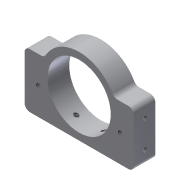
# Autodesk Inventor part: Motor Mount New - Estimated Dimensions
Saved by Autodesk Inventor 2013 (Build 170138000, 138)
## iProperties
Created: 2013-07-20
Part Number: Motor Mount New - Estimated Dimensions
Material: Aluminum 6061
Document SubType Name: Modeling
Designer: Nemo
Density: 1 g/cm^3
Author: Nemo
Autodesk Inventor part; units mm, degrees
ref_plane "YZ Plane" through (0, 0, 0) normal (1, 0, 0) x (0, 1, 0)
ref_plane "XZ Plane" through (0, 0, 0) normal (0, 1, 0) x (-1, 0, 0)
ref_plane "XY Plane" through (0, 0, 0) normal (0, 0, 1) x (1, 0, 0)
sketch "Sketch1" plane through (0, 0, 0) normal (0, 0, 1) x (1, 0, 0)
  circle A0 centre (0, 0) radius 18.5
  line L0 (32, 9.5) -> (32, -22.5)
  line L1 (32, -22.5) -> (-32, -22.5)
  line L2 (-32, -22.5) -> (-32, 9.5)
  arc A1 (20.3961, 9.5) -> (-20.3961, 9.5) centre (0, 0) ccw
  line L3 (-32, 9.5) -> (-20.3961, 9.5)
  line L4 (20.3961, 9.5) -> (32, 9.5)
  point P0 (0, -22.5)
  dimension "d0" = 37
  dimension "d1" = 22.5
  dimension "d2" = 64
  dimension "d3" = 22.5
  dimension "d4" = 32
  constraints: 10 end point, 2 centre point, 2 coincident, 2 horizontal, 2 point on circle, 1 collinear, 1 horizontal alignment, 1 midpoint, 1 parallel, 1 perpendicular, 1 vertical alignment
  measures "d0" diameter of A0
  measures "d1" distance from line of L1 A0.centre
  measures "d2" distance of L0.end L1.end
  measures "d3" radius of A1
  measures "d4" distance between parallel lines of L1 L3
extrude "Extrusion1" add sketch "Sketch1" along normal blind 12.7
fillet "Fillet1" radius 3.175 6 edges at (32, 9.5, 6.35) (20.3961, 9.5, 6.35) (-20.3961, 9.5, 6.35) (-32, 9.5, 6.35) (-32, -22.5, 6.35) (32, -22.5, 6.35)
sketch "Sketch2" plane through (-32, -19.325, 0) normal (-1, 0, 0) x (0, 0, 1)
  line L0 (12.7, -3.175) -> (0, -3.175) projected
  line L1 (0, -3.175) -> (12.7, -3.175) projected
  point P0 (0, 19.325)
  point P1 (6.35, 20.825)
  point P2 (6.35, 4.825)
  point P3 (6.35, 0)
  dimension "d8" = 16
  dimension "d11" = 8
  constraints: 2 vertical alignment
  measures "d8" distance of point (6.35, 4.825) point (6.35, 20.825)
  measures "d11" distance from line of L0 point (6.35, 4.825)
hole "Hole1" at (-32, 1.5, 6.35) at (-32, -14.5, 6.35) direction (1, 0, 0) diameter 2.6416 depth 11.1125 tip angle 118 thread size "6-32 UNC" class "2B" standard "ANSI Unified Screw Threads"
sketch "Sketch4" plane through (-28.825, -22.5, 0) normal (0, -1, 0) x (1, 0, 0)
  line L0 (-3.175, 5.0292) -> (-3.175, 7.6708) projected
  line L1 (-3.175, 5.0292) -> (-3.175, 7.6708) projected
  line L2 (-3.175, 12.7) -> (-3.175, 0) projected
  line L3 (-3.175, 0) -> (-3.175, 12.7) projected
  circle A0 centre (28.825, 6.35) radius 8 construction
  point P0 (20.825, 6.35)
  point P1 (36.825, 6.35)
  point P2 (-3.175, 6.35)
  point P3 (-3.175, 6.35)
  point P4 (-3.175, 6.35)
  point P5 (4.825, 6.35)
  point P6 (52.825, 6.35)
  point P7 (-3.175, 6.35)
  dimension "d24" = 16
  dimension "d19" = 16
  dimension "d23" = 32
  dimension "d43" = 16
  dimension "d44" = 16
  constraints: 6 horizontal alignment, 4 midpoint, 2 other
  measures "d19" distance of point (36.825, 6.35) point (20.825, 6.35)
  measures "d23" distance from line of L2 point (28.825, 6.35)
  measures "d43" distance of point (20.825, 6.35) point (4.825, 6.35)
  measures "d44" distance of point (52.825, 6.35) point (36.825, 6.35)
hole "Hole2" at (-8, -22.5, 6.35) at (8, -22.5, 6.35) at (24, -22.5, 6.35) at (-24, -22.5, 6.35) direction (0, 1, 0) diameter 2.6416 depth 11.1125 tip angle 118 thread size "6-32 UNC" class "2B" standard "ANSI Unified Screw Threads"
mirror "Mirror1" about plane through (0, 0, 0) normal (1, 0, 0) of "Hole1"
sketch "Sketch5" plane through (0, 0, 12.7) normal (0, 0, 1) x (1, 0, 0)
  arc A0 (19.5671, 11.1076) -> (-19.5671, 11.1076) centre (0, 0) ccw projected
  line L0 (-28.825, -22.5) -> (28.825, -22.5) projected
  point P0 (-24, -6.5)
  point P1 (24, -6.5)
  dimension "d32" = 48
  dimension "d34" = 24
  dimension "d35" = 16
  constraints: 1 horizontal alignment
  measures "d32" distance of point (24, -6.5) point (-24, -6.5)
  measures "d34" horizontal distance of A0.centre point (-24, -6.5)
  measures "d35" distance from line of L0 point (-24, -6.5)
hole "Hole3" at (-24, -6.5, 12.7) at (24, -6.5, 12.7) direction (0, 0, -1) diameter 2.6416 end through all thread size "6-32 UNC" class "2B" standard "ANSI Unified Screw Threads"
equation "\"d34\" = 0.5 * d32"
body "Solid1"
